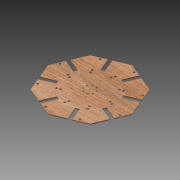
# Autodesk Inventor part: octoBoto01
Saved by Autodesk Inventor 2013 (Build 170138000, 138)
## iProperties
Created: 2014-08-20
Part Number: octoBoto01
Material: Wood (Birch)
Document SubType Name: Modeling
Designer: Nano
Density: 0.55 g/cm^3
Mass: 105.421 g
Surface Area: 1267.67 cm^2
Volume: 191.674 cm^3
Author: Nano
Autodesk Inventor part; units mm, degrees
ref_plane "YZ Plane" through (0, 0, 0) normal (1, 0, 0) x (0, 1, 0)
ref_plane "XZ Plane" through (0, 0, 0) normal (0, 1, 0) x (-1, 0, 0)
ref_plane "XY Plane" through (0, 0, 0) normal (0, 0, 1) x (1, 0, 0)
sketch "Sketch1" plane through (0, 0, 0) normal (0, 1, 0) x (-1, 0, 0)
  line L0 (152.4, 0) -> (107.7631, -107.7631)
  line L1 (107.7631, -107.7631) -> (0, -152.4)
  line L2 (0, -152.4) -> (-107.7631, -107.7631)
  line L3 (-107.7631, -107.7631) -> (-152.4, 0)
  line L4 (-152.4, 0) -> (-107.7631, 107.7631)
  line L5 (-107.7631, 107.7631) -> (0, 152.4)
  line L6 (0, 152.4) -> (107.7631, 107.7631)
  line L7 (107.7631, 107.7631) -> (152.4, 0)
  point P0 (0, 0)
  point P1 (0, 0)
  dimension "d0" = 304.8
  constraints: 16 end point, 17 other
  measures "d0" distance of L0.start L3.end
extrude "Extrusion1" add sketch "Sketch1" along normal blind 3.175
sketch "Sketch2" plane through (0, 3.175, 0) normal (0, 1, 0) x (1, 0, 0)
  line L0 (-152.4, 0) -> (-107.7631, -107.7631) projected
  line L1 (-129.0805, -56.2982) -> (-13.0426, -8.2337) construction
  line L2 (-131.5106, -50.4316) -> (-126.6505, -62.1648)
  line L3 (-126.6505, -62.1648) -> (-79.7174, -42.7245)
  line L4 (-79.7174, -42.7245) -> (-84.5775, -30.9912)
  line L5 (-84.5775, -30.9912) -> (-131.5106, -50.4316)
  point P0 (0, 0)
  dimension "d3" = 6.35
  dimension "d5" = 6.35
  dimension "d6" = 50.8
  constraints: 10 end point, 2 parallel, 1 collinear, 1 perpendicular
  measures "d3" distance of L2.end L1.start
  measures "d5" distance of L2.start L1.start
  measures "d6" distance between parallel lines of L0 L4
extrude "Extrusion2" cut sketch "Sketch2" against normal through all
pattern_circular "Circular Pattern1" count 8 over 360 about axis through (0, -10, 0) along (0, 1, 0) of "Extrusion2"
sketch "Sketch3" plane through (0, 3.175, 0) normal (0, 1, 0) x (1, 0, 0)
  circle A0 centre (0, 0) radius 19.8134 construction
  line L0 (-9.9151, -17.4454) -> (-3.9676, -19.6701)
  line L1 (-3.9676, -19.6701) -> (-2.8552, -16.6963)
  line L2 (-2.8552, -16.6963) -> (-8.8028, -14.4717)
  line L3 (-8.8028, -14.4717) -> (-9.9151, -17.4454)
  line L4 (0, 0) -> (-6.9413, -18.5578) construction
  dimension "d12" = 6.35
  dimension "d14" = 3.175
  dimension "d15" = 3.175
  dimension "d16" = 3.175
  constraints: 10 end point, 2 parallel, 2 perpendicular, 1 centre point, 1 coincident, 1 midpoint, 1 tangent, 1 other
  measures "d12" distance of L1.end L2.end
  measures "d14" distance of L0.end L1.end
  measures "d15" distance of L0.end L4.end
  measures "d16" distance of L0.start L4.end
extrude "Extrusion3" cut sketch "Sketch3" against normal through all
pattern_circular "Circular Pattern2" count 8 over 360 about axis through (0, -10, 0) along (0, 1, 0) of "Extrusion3"
sketch "Sketch4" plane through (0, 3.175, 0) normal (0, 1, 0) x (1, 0, 0)
  line L0 (-4.1298, -90.1076) -> (-1.6998, -84.241) projected
  line L1 (-1.6998, -84.241) -> (-7.5664, -81.8109) projected
  line L2 (-7.5664, -81.8109) -> (-9.9964, -87.6776) projected
  line L3 (-9.9964, -87.6776) -> (-4.1298, -90.1076) projected
  line L4 (0.2443, -79.5477) -> (2.6743, -73.681) projected
  line L5 (2.6743, -73.681) -> (-3.1923, -71.251) projected
  line L6 (-3.1923, -71.251) -> (-5.6224, -77.1176) projected
  line L7 (-5.6224, -77.1176) -> (0.2443, -79.5477) projected
  line L8 (-24.224, -138.6194) -> (-21.794, -132.7528) projected
  line L9 (-21.794, -132.7528) -> (-27.6606, -130.3227) projected
  line L10 (-27.6606, -130.3227) -> (-30.0907, -136.1894) projected
  line L11 (-30.0907, -136.1894) -> (-24.224, -138.6194) projected
  point P0 (0, 0)
extrude "Extrusion4" cut sketch "Sketch4" against normal through all
pattern_circular "Circular Pattern3" count 8 over 360 about axis through (0, -10, 0) along (0, 1, 0) of "Extrusion4"
sketch "Sketch5" plane through (0, 3.175, 0) normal (0, 1, 0) x (1, 0, 0)
  circle A0 centre (0, 0) radius 1.5875
  circle A1 centre (-35.8781, -30.9912) radius 1.5875
  circle A2 centre (44.7782, -15.5757) radius 1.5875
  circle A3 centre (-8.9002, 46.567) radius 1.5875
  dimension "d27" = 3.175
  dimension "d28" = 3.175
  dimension "d31" = 360
  constraints: 4 centre point, 7 other
  measures "d27" diameter of A0
  measures "d28" diameter of A1
extrude "Extrusion5" cut sketch "Sketch5" against normal through all
equation "\"d5\" = d3"
equation "\"d15\" = d16"
body "Solid1"
